Autodesk Fusion 360 part; units mm, degrees
note: some values were not read from the file. Set by a fixed rule: which face or edge a step refers to.
(part 2 of 2)
extrude "Extrude13" add sketch "roof_wall2" along normal up to surface (1 mm away) contours L1 L2 L3 L10 L11 L12 L13 L14 L15 L16 L17 L18 L19 bodies 2
extrude "Extrude14" cut sketch "roof_high" along normal up to surface (3 mm away) contours L1 L4 L8 L32 L33 L34 L35 L36 | L1 L32 L36 L37 L38 L39 bodies 2
extrude "Extrude15" cut sketch "roof_high" against normal up to surface (5.7 mm away) contours L1 L4 L8 L32 L33 L34 L35 L36 bodies 2
fillet "Fillet1" radius 1 1 faces at (-22.7917, -2.845, 19) on bodies 2
fillet "Fillet2" radius 1 1 faces at (2.525, 43.415, 10.3) on bodies 2
fillet "Fillet3" radius 1 1 edges at (0.025, 35.315, 16) on bodies 2
fillet "Fillet4" radius 1 1 edges at (0.025, -44.365, 15) on bodies 2
sketch "case_floor" plane through (0, 0, 0) normal (0, 0, -1) x (1, 0, 0)
  line L0 (1.8, 41.415) -> (20.9, 41.415)
  line L1 (27.5, 41.415) -> (27.5, -41.415)
  line L2 (27.5, -41.415) -> (-27.5, -41.415)
  line L3 (-30.45, -44.415) -> (30.5, -44.415)
  line L4 (30.5, -44.415) -> (30.5, 44.365)
  line L5 (30.5, 44.365) -> (-30.45, 44.365)
  line L6 (-30.45, 44.365) -> (-30.45, -44.415)
  line L7 (30.5, -44.415) -> (-30.45, -44.415)
  line L8 (-30.45, -44.415) -> (-30.45, 44.365)
  line L9 (-30.45, 44.365) -> (30.5, 44.365)
  line L10 (30.5, 44.365) -> (30.5, -44.415)
  line L11 (-24.5, 41.415) -> (-24.5, 42.915)
  line L12 (-24.5, 42.915) -> (-20.9, 42.915)
  line L13 (-20.9, 42.915) -> (-20.9, 41.415)
  line L14 (20.9, 41.415) -> (20.9, 42.915)
  line L15 (20.9, 42.915) -> (24.5, 42.915)
  line L16 (24.5, 42.915) -> (24.5, 41.415)
  line L17 (-27.5, -41.415) -> (-27.5, -28.915)
  line L18 (-27.5, -28.915) -> (-29, -28.915)
  line L19 (-29, -28.915) -> (-29, -25.315)
  line L20 (-29, -25.315) -> (-27.5, -25.315)
  line L21 (-27.5, 24.815) -> (-29, 24.815)
  line L22 (-29, 24.815) -> (-29, 28.415)
  line L23 (-29, 28.415) -> (-27.5, 28.415)
  line L24 (-27.5, 41.415) -> (-24.5, 41.415)
  line L25 (-20.9, 41.415) -> (-1.8, 41.415)
  line L26 (-1.8, 41.415) -> (-1.8, 42.915)
  line L27 (-1.8, 42.915) -> (1.8, 42.915)
  line L28 (1.8, 42.915) -> (1.8, 41.415)
  line L29 (-27.5, 28.415) -> (-27.5, 41.415)
  line L30 (24.5, 41.415) -> (27.5, 41.415)
  line L31 (-27.5, 41.415) -> (-30.45, 41.415) construction
  line L32 (-30.45, 41.415) -> (-30.45, 29.415)
  line L33 (27.5, -41.415) -> (27.5, 41.415) construction
  line L34 (20.9, 41.415) -> (1.8, 41.415) construction
  line L35 (-27.5, -41.415) -> (27.5, -41.415) construction
  line L36 (27.5, 41.415) -> (30.5, 41.415) construction
  line L37 (-27.5, -41.415) -> (-30.45, -41.415) construction
  line L38 (27.5, -41.415) -> (30.5, -41.415) construction
  circle A0 centre (33.5, -35.415) radius 6
  circle A1 centre (33.5, -35.415) radius 1.65
  circle A2 centre (33.5, -35.415) radius 1.35
  circle A3 centre (33.5, 35.415) radius 6
  circle A4 centre (33.5, 35.415) radius 1.65
  circle A5 centre (33.5, 35.415) radius 1.35
  circle A6 centre (-33.5, 35.415) radius 6
  circle A7 centre (-33.5, 35.415) radius 1.65
  circle A8 centre (-33.5, 35.415) radius 1.35
  circle A9 centre (-33.5, -35.415) radius 6
  circle A10 centre (-33.5, -35.415) radius 1.65
  circle A11 centre (-33.5, -35.415) radius 1.35
  dimension "d184" = 12
  dimension "d185" = 2.7
  dimension "d186" = 3.3
  dimension "d187" = 12
  dimension "d188" = 2.7
  dimension "d189" = 3.3
  dimension "d190" = 12
  dimension "d191" = 2.7
  dimension "d192" = 3.3
  dimension "d193" = 12
  dimension "d194" = 3.3
  dimension "d195" = 2.7
  constraint horizontal L7
  constraint vertical L8
  constraint horizontal L9
  constraint coincident L5.end L6.start
  constraint coincident L3.end L4.start
  constraint coincident L24.start L29.end
  constraint coincident L8 L31.end
  constraint perpendicular L8 L31
  constraint coincident L8 L32.end
  constraint coincident L1.start L30.end
  constraint coincident L10 L36.end
  constraint perpendicular L10 L36
  constraint coincident L2.end L17.start
  constraint coincident L8 L37.end
  constraint perpendicular L8 L37
  constraint coincident L1.end L2.start
  constraint coincident L10 L38.end
  constraint perpendicular L10 L38
  constraint tangent L38 A0
  constraint tangent L1 A0
  constraint concentric A0 A1
  constraint concentric A0 A2
  constraint tangent L36 A3
  constraint tangent L1 A3
  constraint concentric A3 A4
  constraint concentric A4 A5
  constraint tangent L31 A6
  constraint tangent L29 A6
  constraint concentric A6 A7
  constraint concentric A7 A8
  constraint tangent L37 A9
  constraint tangent L17 A9
  constraint concentric A9 A10
  constraint concentric A10 A11
  measures "d184" diameter of A0
  measures "d185" diameter of A2
  measures "d186" diameter of A1
  measures "d187" diameter of A3
  measures "d188" diameter of A5
  measures "d189" diameter of A4
  measures "d190" diameter of A6
  measures "d191" diameter of A8
  measures "d192" diameter of A7
  measures "d193" diameter of A9
  measures "d194" diameter of A10
  measures "d195" diameter of A11
extrude "Extrude5" add sketch "case_floor" along normal blind 3 separate body contours L0 L1 L4 L5 L6 L8 L9 L10 L11 L12 L13 L14 L15 L16 L24 L25 L26 L27 L28 L29 L30 L32 A3 A6 | L0 L1 L2 L6 L8 L11 L12 L13 L14 L15 L16 L17 L24 L25 L26 L27 L28 L29 L30 L32 A6 A9 | L1 L4 L10 A0 A3 | L4 L10 A3 | L1 L2 L3 L4 L6 L7 L8 L10 L17 A0 A9 | L4 L10 A0 | L4 L10 A3 | L4 L10 A0 | L6 L8 L32 A6 | L6 L8 A9 | L6 L8 L32 A6 | L6 L8 A9 makes body 3
extrude "Extrude17" add sketch "case_floor" against normal blind 7.3 contours L4 L10 A3 | L4 L10 A0 | L6 L8 L32 A6 | L6 L8 A9 | A1 | A4 | A7 | A10 picked at (30.95, 35.415) picked at (30.95, -35.415) picked at (-30.9167, 35.415) picked at (-30.9167, -35.415) bodies 2
sketch "boss" plane through (0, 0, 7.3) normal (0, 0, 1) x (-1, 0, 0)
  circle A0 centre (33.5, -35.415) radius 6
  circle A1 centre (-33.5, -35.415) radius 6
  circle A2 centre (-33.5, 35.415) radius 6
  circle A3 centre (33.5, 35.415) radius 6
extrude "Extrude18" add sketch "boss" along normal blind 1.5 bodies 2
sketch "leg1" plane through (0, 0, -3) normal (0, 0, -1) x (1, 0, 0)
  line L0 (-30.45, 30.248) -> (-30.45, -30.248)
  line L1 (-30.45, -44.415) -> (30.5, -44.415)
  line L2 (30.5, -44.415) -> (30.5, -40.6112)
  line L3 (30.5, 44.365) -> (-30.45, 44.365)
  line L4 (-30.45, -30.248) -> (30.5, 44.365) construction
  line L5 (30.5, -44.415) -> (-30.45, 44.365) construction
  line L6 (0.025, 44.365) -> (0.025, -44.415) construction
  line L7 (30.5, 0) -> (-30.45, 0) construction
  circle A0 centre (-25.45, 0) radius 3
  circle A1 centre (25.5, -0.0125) radius 3
  circle A2 centre (0.025, 39.365) radius 3
  circle A3 centre (0.025, -39.415) radius 3
  arc A4 (-30.45, 40.582) -> (-30.45, 30.248) centre (-33.5, 35.415) ccw
  line L8 (-30.45, 44.365) -> (-30.45, 40.582)
  line L9 (-30.45, -40.582) -> (-30.45, -44.415)
  line L10 (30.5, -30.2188) -> (30.5, 30.2188)
  line L11 (30.5, 40.6112) -> (30.5, 44.365)
  circle A5 centre (-33.5, 35.415) radius 1.65
  circle A6 centre (33.5, -35.415) radius 1.65
  circle A7 centre (-33.5, -35.415) radius 1.65
  circle A8 centre (33.5, 35.415) radius 1.65
  arc A9 (30.5, -40.6112) -> (30.5, -30.2188) centre (33.5, -35.415) ccw
  arc A10 (30.5, 30.2188) -> (30.5, 40.6112) centre (33.5, 35.415) ccw
  arc A11 (-30.45, -30.248) -> (-30.45, -40.582) centre (-33.5, -35.415) ccw
  dimension "d160" = 6
  dimension "d161" = 6
  dimension "d162" = 6
  dimension "d163" = 6
  dimension "d164" = 5
  dimension "d166" = 5
  constraint coincident L0.end L4.start
  constraint coincident L3.start L4.end
  constraint coincident L1.end L2.start
  constraint coincident L3.end L5.end
  constraint midpoint L3 L6.start
  constraint midpoint L1 L6.end
  measures "d160" diameter of A0
  measures "d161" diameter of A1
  measures "d162" diameter of A3
  measures "d163" diameter of A2
  measures "d164" distance of L3 A2.centre
  measures "d166" distance of L1 A3.centre
ref_plane "WorkPlane4" through (-0.0106, 0.025, -6) normal (0, 0, -1) x (1, 0, 0)
sketch "leg2" plane through (0, 0, -6) normal (0, 0, -1) x (-1, 0, 0)
  circle A0 centre (-25.5, 0.0125) radius 3
  circle A1 centre (25.45, 0) radius 3
  circle A2 centre (-0.025, -39.365) radius 3
  circle A3 centre (-0.025, 39.415) radius 3
  circle A4 centre (-0.025, 39.415) radius 4.5
  circle A5 centre (-25.5, 0.0125) radius 4.5
  circle A6 centre (-0.025, -39.365) radius 4.5
  circle A7 centre (25.45, 0) radius 4.5
  dimension "d168" = 9
  dimension "d169" = 9
  dimension "d170" = 9
  dimension "d171" = 9
  constraint concentric A3 A4
  constraint concentric A0 A5
  constraint concentric A2 A6
  constraint concentric A1 A7
  measures "d168" diameter of A7
  measures "d169" diameter of A6
  measures "d170" diameter of A4
  measures "d171" diameter of A5
loft "Loft1" add profiles "leg1", "leg2" section 1 contours A1 section 2 contours A0 | A5 bodies 3
loft "Loft2" add profiles "leg1", "leg2" section 1 contours A3 section 2 contours A3 | A4 bodies 3
loft "Loft3" add profiles "leg1", "leg2" section 1 contours A0 section 2 contours A1 | A7 bodies 3
loft "Loft4" add profiles "leg1", "leg2" section 1 contours A2 section 2 contours A2 | A6 bodies 3
fillet "Fillet6" radius 1 20 edges at (-30.45, -40.582, 4.4) (-30.45, -35.415, 8.8) (-30.45, -30.248, 4.4) (-30.45, 40.582, 4.4) (-30.45, 35.415, 8.8) (-30.45, 30.248, 4.4) (30.5, 30.2188, 4.4) (30.5, 35.415, 8.8) (30.5, 40.6112, 4.4) (30.5, -35.415, 8.8) (30.5, -40.6112, 4.4) (30.5, -30.2188, 4.4) (-30.45, -30.248, -1.5) (-30.45, -40.582, -1.5) (-30.45, 30.248, -1.5) (-30.45, 40.582, -1.5) (30.5, 30.2188, -1.5) (30.5, 40.6112, -1.5) (30.5, -40.6112, -1.5) (30.5, -30.2188, -1.5) on bodies 2 3
hidden bodies 1
equation "d1 = board_width"
equation "d2 = board_length"
equation "d5 = d2 / 2"
equation "d7 = d1 / 2"
equation "d8 = board_height"
equation "ravine_width = ravine_wdith"
equation "pin_spacing = 0.1 in"
equation "d35 = pin_spacing * 4"
equation "d36 = -pin_spacing * 14"
equation "d40 = pin_spacing"
equation "d41 = 2 * pin_spacing"
equation "d45 = 12 * pin_spacing"
equation "board_width = 54.4 mm"
equation "board_length = 82.23 mm"
equation "board_height = 10 mm"
equation "d59 = tolerance"
equation "d61 = case_width"
equation "d62 = case_width"
equation "d66 = -board_height - tolerance - rasberry_pi_height"
equation "d68 = case_width"
equation "case_width = 3 mm"
equation "ravine_wdith = 3 mm"
equation "d85 = ravine_wdith"
equation "d87 = ravine_wdith"
equation "d90 = ravine_wdith"
equation "d94 = ravine_wdith"
equation "tolerance = 0.3 mm"
equation "peg_height = 5 mm"
equation "d97 = tolerance"
equation "rasberry_pi_height = 5.7 mm"
equation "d101 = rasberry_pi_length"
equation "rasberry_pi_length = 53 mm"
equation "d106 = case_width"
equation "d117 = tolerance"
equation "d155 = -7.00 mm - tolerance"
named bodies: "breadboard_body", "case_base", "case_floor"
